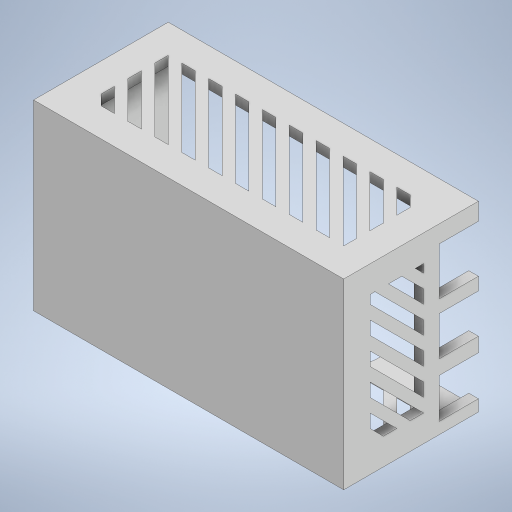
# Autodesk Inventor part: RPIcaseTop
Saved by Autodesk Inventor 2024 (Build 280153000, 153)
## iProperties
Created: 2023-07-18
Part Number: RPIcaseTop
Material: Generic
Document SubType Name: Modeling
Designer: 18179
Density: 1 g/cm^3
Appearance: Default
Autodesk Inventor part; units mm, degrees
ref_plane "YZ Plane" through (0, 0, 0) normal (1, 0, 0) x (0, 1, 0)
ref_plane "XZ Plane" through (0, 0, 0) normal (0, 1, 0) x (-1, 0, 0)
ref_plane "XY Plane" through (0, 0, 0) normal (0, 0, 1) x (1, 0, 0)
sketch "Sketch1" plane through (0, 0, 0) normal (0, 0, 1) x (1, 0, 0)
  point P0 (0, 0)
sketch "0" plane through (0, 0, 0) normal (0, 0, 1) x (1, 0, 0)
  line L0 (-14.825, -56.3549) -> (-14.825, 0.3263)
  line L1 (-14.825, 0.3263) -> (82.381, 0.3263)
  line L2 (82.381, 0.3263) -> (82.381, -2.3)
  line L3 (82.381, -2.3) -> (85.6, -2.3)
  line L4 (85.6, -2.3) -> (85.6, 3.5013)
  line L5 (85.6, 3.5013) -> (-18, 3.5013)
  line L6 (-18, 3.5013) -> (-18, -57.5)
  line L7 (-18, -57.5) -> (3.4071, -57.5)
  line L8 (3.4071, -57.5) -> (3.4071, -56.3549)
  line L9 (3.4071, -56.3549) -> (-14.825, -56.3549)
  line L10 (-14.825, -56.3549) -> (82.381, -56.3549)
  line L11 (82.381, -56.3549) -> (82.381, 0.3263)
  line L12 (82.381, 0.3263) -> (-14.825, 0.3263)
  line L13 (-14.825, 0.3263) -> (-14.825, -56.3549)
  line L14 (13.029, -57.5) -> (13.029, -56.3549)
  line L15 (13.029, -56.3549) -> (3.4071, -56.3549)
  line L16 (3.4071, -56.3549) -> (3.4071, -57.5)
  line L17 (3.4071, -57.5) -> (13.029, -57.5)
  line L18 (19.369, -56.3549) -> (13.029, -56.3549)
  line L19 (13.029, -56.3549) -> (13.029, -57.5)
  line L20 (13.029, -57.5) -> (19.369, -57.5)
  line L21 (19.369, -57.5) -> (19.369, -56.3549)
  line L22 (26.631, -57.5) -> (26.631, -56.3549)
  line L23 (26.631, -56.3549) -> (19.369, -56.3549)
  line L24 (19.369, -56.3549) -> (19.369, -57.5)
  line L25 (19.369, -57.5) -> (26.631, -57.5)
  line L26 (32.869, -56.3549) -> (26.631, -56.3549)
  line L27 (26.631, -56.3549) -> (26.631, -57.5)
  line L28 (26.631, -57.5) -> (32.869, -57.5)
  line L29 (32.869, -57.5) -> (32.869, -56.3549)
  line L30 (40.131, -57.5) -> (40.131, -56.3549)
  line L31 (40.131, -56.3549) -> (32.869, -56.3549)
  line L32 (32.869, -56.3549) -> (32.869, -57.5)
  line L33 (32.869, -57.5) -> (40.131, -57.5)
  line L34 (47.619, -56.3549) -> (40.131, -56.3549)
  line L35 (40.131, -56.3549) -> (40.131, -57.5)
  line L36 (40.131, -57.5) -> (47.619, -57.5)
  line L37 (47.619, -57.5) -> (47.619, -56.3549)
  line L38 (54.381, -57.5) -> (54.381, -56.3549)
  line L39 (54.381, -56.3549) -> (47.619, -56.3549)
  line L40 (47.619, -56.3549) -> (47.619, -57.5)
  line L41 (47.619, -57.5) -> (54.381, -57.5)
  line L42 (82.381, -56.3549) -> (54.381, -56.3549)
  line L43 (54.381, -56.3549) -> (54.381, -57.5)
  line L44 (54.381, -57.5) -> (85.6, -57.5)
  line L45 (85.6, -57.5) -> (85.6, -53.65)
  line L46 (85.6, -53.65) -> (82.381, -53.65)
  line L47 (82.381, -53.65) -> (82.381, -56.3549)
  line L48 (82.381, -53.65) -> (85.6, -53.65)
  line L49 (85.6, -53.65) -> (85.6, -40.35)
  line L50 (85.6, -40.35) -> (82.381, -40.35)
  line L51 (82.381, -40.35) -> (82.381, -53.65)
  line L52 (82.381, -35.55) -> (85.6, -35.55)
  line L53 (85.6, -35.55) -> (85.6, -22.45)
  line L54 (85.6, -22.45) -> (82.381, -22.45)
  line L55 (82.381, -22.45) -> (82.381, -35.55)
  line L56 (82.381, -18.2) -> (85.6, -18.2)
  line L57 (85.6, -18.2) -> (85.6, -2.3)
  line L58 (85.6, -2.3) -> (82.381, -2.3)
  line L59 (82.381, -2.3) -> (82.381, -18.2)
  line L60 (85.6, -18.2) -> (82.381, -18.2)
  line L61 (82.381, -18.2) -> (82.381, -22.45)
  line L62 (82.381, -22.45) -> (85.6, -22.45)
  line L63 (85.6, -22.45) -> (85.6, -18.2)
  line L64 (85.6, -40.35) -> (85.6, -35.55)
  line L65 (85.6, -35.55) -> (82.381, -35.55)
  line L66 (82.381, -35.55) -> (82.381, -40.35)
  line L67 (82.381, -40.35) -> (85.6, -40.35)
  circle A0 centre (58.5, -3.5) radius 1.35
  circle A1 centre (58.5, -52.5) radius 1.35
  circle A2 centre (0.5, -52.5) radius 1.35
  circle A3 centre (0.5, -3.5) radius 1.35
  line L68 (26.631, -57.5) -> (32.869, -57.5)
  line L69 (85.6, -18.2) -> (85.6, -2.3)
  point P0 (-14.825, 0.3263)
  point P1 (82.381, -2.3)
  point P2 (85.6, 3.5013)
  point P3 (-18, 3.5013)
  constraints: 140 end point, 4 centre point
extrude "Extrusion1" add sketch "0" along normal blind 40 contours L9 L8 L7 L6 L5 L4 L3 L2 L1 L0 | L10 L21 L20 L14 | L56 L63 L54 L11 | L10 L29 L28 L22 | L52 L64 L50 L11 | L10 L37 L36 L30 | L46 L45 L44 L38 L10 L11
sketch "Sketch3" plane through (0, 0, 40) normal (0, 0, 1) x (1, 0, 0)
  line L0 (3.4071, -57.5) -> (3.4071, -56.3549) projected
  line L1 (3.4071, -56.3549) -> (-14.825, -56.3549) projected
  line L2 (-14.825, -56.3549) -> (-14.825, 0.3263) projected
  line L3 (-14.825, 0.3263) -> (82.381, 0.3263) projected
  line L4 (82.381, 0.3263) -> (82.381, -2.3) projected
  line L5 (82.381, -2.3) -> (85.6, -2.3) projected
  line L6 (85.6, -2.3) -> (85.6, 3.5013) projected
  line L7 (85.6, 3.5013) -> (-18, 3.5013) projected
  line L8 (-18, 3.5013) -> (-18, -57.5) projected
  line L9 (-18, -57.5) -> (3.4071, -57.5) projected
  line L10 (19.369, -57.5) -> (19.369, -56.3549) projected
  line L11 (19.369, -56.3549) -> (13.029, -56.3549) projected
  line L12 (13.029, -56.3549) -> (13.029, -57.5) projected
  line L13 (13.029, -57.5) -> (19.369, -57.5) projected
  line L14 (40.131, -56.3549) -> (40.131, -57.5) projected
  line L15 (82.381, -56.3549) -> (54.381, -56.3549) projected
  line L16 (32.869, -57.5) -> (32.869, -56.3549) projected
  line L17 (85.6, -57.5) -> (85.6, -53.65) projected
  line L18 (85.6, -53.65) -> (82.381, -53.65) projected
  line L19 (82.381, -53.65) -> (82.381, -56.3549) projected
  line L20 (82.381, -56.3549) -> (54.381, -56.3549) projected
  line L21 (47.619, -57.5) -> (47.619, -56.3549) projected
  line L22 (85.6, -35.55) -> (82.381, -35.55) projected
  line L23 (82.381, -35.55) -> (82.381, -40.35) projected
  line L24 (82.381, -40.35) -> (85.6, -40.35) projected
  line L25 (85.6, -40.35) -> (85.6, -35.55) projected
  line L26 (85.6, -18.2) -> (82.381, -18.2) projected
  line L27 (82.381, -18.2) -> (82.381, -22.45) projected
  line L28 (82.381, -22.45) -> (85.6, -22.45) projected
  line L29 (85.6, -22.45) -> (85.6, -18.2) projected
  line L30 (-18, -57.5) -> (3.4071, -57.5) projected
  line L31 (3.4071, -57.5) -> (13.029, -57.5)
  line L32 (13.029, -57.5) -> (13.029, -56.3549)
  line L33 (13.029, -56.3549) -> (3.4071, -56.3549)
  line L34 (3.4071, -56.3549) -> (3.4071, -57.5)
  line L35 (19.369, -57.5) -> (32.869, -57.5)
  line L36 (32.869, -57.5) -> (32.869, -56.3549)
  line L37 (32.869, -56.3549) -> (19.369, -56.3549)
  line L38 (19.369, -56.3549) -> (19.369, -57.5)
  line L39 (40.131, -57.5) -> (47.619, -57.5)
  line L40 (47.619, -57.5) -> (47.619, -56.3549)
  line L41 (47.619, -56.3549) -> (40.131, -56.3549)
  line L42 (40.131, -56.3549) -> (40.131, -57.5)
  line L43 (85.6, -53.65) -> (82.381, -53.65)
  line L44 (82.381, -53.65) -> (82.381, -40.35)
  line L45 (82.381, -40.35) -> (85.6, -40.35)
  line L46 (85.6, -40.35) -> (85.6, -53.65)
  line L47 (85.6, -35.55) -> (82.381, -35.55)
  line L48 (82.381, -35.55) -> (82.381, -22.45)
  line L49 (82.381, -22.45) -> (85.6, -22.45)
  line L50 (85.6, -22.45) -> (85.6, -35.55)
  line L51 (85.6, -18.2) -> (82.381, -18.2)
  line L52 (82.381, -18.2) -> (82.381, -2.3)
  line L53 (82.381, -2.3) -> (85.6, -2.3)
  line L54 (85.6, -2.3) -> (85.6, -18.2)
  line L55 (47.619, -56.3549) -> (40.131, -56.3549) projected
  line L56 (40.131, -56.3549) -> (40.131, -57.5) projected
  line L57 (40.131, -57.5) -> (47.619, -57.5) projected
  line L58 (19.369, -57.5) -> (19.369, -56.3549) projected
  line L59 (19.369, -56.3549) -> (13.029, -56.3549) projected
  line L60 (13.029, -56.3549) -> (13.029, -57.5) projected
  line L61 (13.029, -57.5) -> (19.369, -57.5) projected
  line L62 (32.869, -56.3549) -> (26.631, -56.3549) projected
  line L63 (26.631, -56.3549) -> (26.631, -57.5) projected
  line L64 (26.631, -57.5) -> (32.869, -57.5) projected
  line L65 (32.869, -57.5) -> (32.869, -56.3549) projected
  line L66 (54.381, -56.3549) -> (54.381, -57.5) projected
  line L67 (54.381, -57.5) -> (85.6, -57.5) projected
  line L68 (47.619, -57.5) -> (47.619, -56.3549) projected
  line L69 (47.619, -56.3549) -> (40.131, -56.3549) projected
  line L70 (40.131, -57.5) -> (47.619, -57.5) projected
  line L71 (19.369, -57.5) -> (19.369, -56.3549) projected
  line L72 (19.369, -56.3549) -> (13.029, -56.3549) projected
  line L73 (13.029, -56.3549) -> (13.029, -57.5) projected
  line L74 (13.029, -57.5) -> (19.369, -57.5) projected
  line L75 (32.869, -56.3549) -> (26.631, -56.3549) projected
  line L76 (26.631, -56.3549) -> (26.631, -57.5) projected
  line L77 (26.631, -57.5) -> (32.869, -57.5) projected
  line L78 (85.6, -53.65) -> (82.381, -53.65) projected
  line L79 (82.381, -53.65) -> (82.381, -56.3549) projected
  line L80 (54.381, -56.3549) -> (54.381, -57.5) projected
  line L81 (54.381, -57.5) -> (85.6, -57.5) projected
  line L82 (85.6, -57.5) -> (85.6, -53.65) projected
  point P0 (0, 0)
  constraints: 48 end point, 12 parallel, 6 horizontal, 6 perpendicular
extrude "Extrusion2" add sketch "Sketch3" against normal blind 26.919 contours L54 L26 L52 L5 | L50 L22 L48 L28 | L46 L18 L44 L24
sketch "Sketch6" plane through (0, 0, 40) normal (0, 0, 1) x (1, 0, 0)
  line L0 (54.381, -56.3549) -> (54.381, -57.5) projected
  line L1 (47.619, -56.3549) -> (40.131, -56.3549) projected
  line L2 (54.381, -57.5) -> (47.619, -57.5)
  line L3 (47.619, -57.5) -> (47.619, -56.3549)
  line L4 (47.619, -56.3549) -> (54.381, -56.3549)
  line L5 (54.381, -56.3549) -> (54.381, -57.5)
  point P0 (0, 0)
  constraints: 8 end point, 2 parallel, 1 horizontal, 1 perpendicular
extrude "Extrusion4" add sketch "Sketch6" against normal blind 33.2436
fillet "Fillet2" radius 3.175 2 edges at (47.619, -56.9275, 6.7564) (54.381, -56.9275, 6.7564)
sketch "Sketch7" plane through (0, 0, 40) normal (0, 0, 1) x (1, 0, 0)
  line L0 (3.4071, -57.5) -> (3.4071, -56.3549) projected
  line L1 (13.029, -57.5) -> (19.369, -57.5) projected
  line L2 (3.4071, -56.3549) -> (13.029, -56.3549)
  line L3 (13.029, -56.3549) -> (13.029, -57.5)
  line L4 (13.029, -57.5) -> (3.4071, -57.5)
  line L5 (3.4071, -57.5) -> (3.4071, -56.3549)
  line L6 (19.369, -57.5) -> (19.369, -56.3549) projected
  line L7 (26.631, -56.3549) -> (26.631, -57.5) projected
  line L8 (19.369, -56.3549) -> (26.631, -56.3549)
  line L9 (26.631, -56.3549) -> (26.631, -57.5)
  line L10 (26.631, -57.5) -> (19.369, -57.5)
  line L11 (19.369, -57.5) -> (19.369, -56.3549)
  line L12 (32.869, -57.5) -> (32.869, -56.3549) projected
  line L13 (40.131, -56.3549) -> (40.131, -57.5) projected
  line L14 (32.869, -56.3549) -> (40.131, -56.3549)
  line L15 (40.131, -56.3549) -> (40.131, -57.5)
  line L16 (40.131, -57.5) -> (32.869, -57.5)
  line L17 (32.869, -57.5) -> (32.869, -56.3549)
  point P0 (0, 0)
  constraints: 24 end point, 6 parallel, 3 horizontal, 3 perpendicular
extrude "Extrusion5" add sketch "Sketch7" against normal blind 36.8504
fillet "Fillet3" radius 1.524 2 edges at (3.4071, -56.9275, 3.1496) (13.029, -56.9275, 3.1496)
fillet "Fillet4" radius 0.762 4 edges at (19.369, -56.9275, 3.1496) (26.631, -56.9275, 3.1496) (32.869, -56.9275, 3.1496) (40.131, -56.9275, 3.1496)
sketch "Sketch8" plane through (0, 0, 40) normal (0, 0, 1) x (1, 0, 0)
  line L0 (-14.825, -56.3549) -> (-14.825, 0.3263) projected
  line L1 (-14.825, 0.3263) -> (82.381, 0.3263) projected
  line L2 (82.381, 0.3263) -> (82.381, -56.3549) projected
  line L3 (82.381, -56.3549) -> (-14.825, -56.3549) projected
  point P0 (0, 0)
extrude "Extrusion6" add sketch "Sketch8" against normal blind 2
sketch "Sketch9" plane through (0, 0, 40) normal (0, 0, 1) x (1, 0, 0)
  line L0 (-18, -57.5) -> (85.6, -57.5) projected
  line L1 (85.6, -57.5) -> (85.6, 3.5013) projected
  line L2 (85.6, 3.5013) -> (-18, 3.5013) projected
  line L3 (-18, 3.5013) -> (-18, -57.5) projected
  point P0 (0, 0)
extrude "Extrusion7" add sketch "Sketch9" along normal blind 5
sketch "Sketch10" plane through (54.381, -57.5, 0) normal (0, -1, 0) x (1, 0, 0)
  line L0 (-27.75, 0) -> (-21.512, 0) projected
  line L1 (-21.512, 0) -> (-21.512, 2.3876) projected
  arc A0 (-20.75, 3.1496) -> (-21.512, 2.3876) centre (-20.75, 2.3876) ccw projected
  line L2 (-15.012, 3.1496) -> (-20.75, 3.1496) projected
  arc A1 (-14.25, 2.3876) -> (-15.012, 3.1496) centre (-15.012, 2.3876) ccw projected
  line L3 (-14.25, 0) -> (-14.25, 2.3876) projected
  line L4 (-14.25, 0) -> (-6.762, 0) projected
  line L5 (-6.762, 0) -> (-6.762, 3.5814) projected
  arc A2 (-3.587, 6.7564) -> (-6.762, 3.5814) centre (-3.587, 3.5814) ccw projected
  line L6 (-3.175, 6.7564) -> (-3.587, 6.7564) projected
  arc A3 (0, 3.5814) -> (-3.175, 6.7564) centre (-3.175, 3.5814) ccw projected
  line L7 (0, 0) -> (0, 3.5814) projected
  line L8 (0, 0) -> (31.219, 0) projected
  line L9 (31.219, 0) -> (31.219, 45) projected
  line L10 (-72.381, 45) -> (31.219, 45) projected
  line L11 (-72.381, 0) -> (-72.381, 45) projected
  line L12 (-72.381, 0) -> (-50.9739, 0) projected
  line L13 (-50.9739, 0) -> (-50.9739, 1.6256) projected
  arc A4 (-49.4499, 3.1496) -> (-50.9739, 1.6256) centre (-49.4499, 1.6256) ccw projected
  line L14 (-42.876, 3.1496) -> (-49.4499, 3.1496) projected
  arc A5 (-41.352, 1.6256) -> (-42.876, 3.1496) centre (-42.876, 1.6256) ccw projected
  line L15 (-41.352, 0) -> (-41.352, 1.6256) projected
  line L16 (-41.352, 0) -> (-35.012, 0) projected
  line L17 (-35.012, 0) -> (-35.012, 2.3876) projected
  arc A6 (-34.25, 3.1496) -> (-35.012, 2.3876) centre (-34.25, 2.3876) ccw projected
  line L18 (-28.512, 3.1496) -> (-34.25, 3.1496) projected
  arc A7 (-27.75, 2.3876) -> (-28.512, 3.1496) centre (-28.512, 2.3876) ccw projected
  line L19 (-27.75, 0) -> (-27.75, 2.3876) projected
  line L20 (36.8849, 50.6659) -> (36.8849, -5.6659)
  line L21 (36.8849, -5.6659) -> (-1.0961, -5.6659)
  line L22 (-1.0961, -5.6659) -> (-15.8461, -5.6659)
  line L23 (-15.8461, -5.6659) -> (-29.3461, -5.6659)
  line L24 (-29.3461, -5.6659) -> (-45.3079, -5.6659)
  line L25 (-45.3079, -5.6659) -> (-78.0469, -5.6659)
  line L26 (-78.0469, -5.6659) -> (-78.0469, 50.6659)
  line L27 (-78.0469, 50.6659) -> (36.8849, 50.6659)
  line L28 (21.6449, 35.4259) -> (21.6449, 9.5741)
  line L29 (21.6449, 9.5741) -> (-1.0961, 9.5741)
  line L30 (-1.0961, 9.5741) -> (-15.8461, 9.5741)
  line L31 (-15.8461, 9.5741) -> (-29.3461, 9.5741)
  line L32 (-29.3461, 9.5741) -> (-45.3079, 9.5741)
  line L33 (-45.3079, 9.5741) -> (-62.8069, 9.5741)
  line L34 (-62.8069, 9.5741) -> (-62.8069, 35.4259)
  line L35 (-62.8069, 35.4259) -> (21.6449, 35.4259)
  line L36 (-62.8069, 9.5741) -> (-34.25, 38.131)
  line L37 (-62.8069, 9.5741) -> (-22.4213, 9.5741) construction
  line L38 (-60.5619, 7.329) -> (-32.0049, 35.8859)
  line L39 (-58.3168, 5.0839) -> (-29.7599, 33.6409)
  line L40 (-65.052, 11.8191) -> (-36.4951, 40.3761)
  line L41 (-67.2971, 14.0642) -> (-38.7401, 42.6211)
  line L42 (-69.5421, 16.3092) -> (-40.9852, 44.8662)
  line L43 (-71.7872, 18.5543) -> (-43.2303, 47.1113)
  line L44 (-74.0323, 20.7994) -> (-45.4753, 49.3563)
  line L45 (-56.0718, 2.8389) -> (-27.5148, 31.3958)
  line L46 (-53.8267, 0.5938) -> (-25.2697, 29.1507)
  line L47 (-51.5816, -1.6513) -> (-23.0247, 26.9057)
  line L48 (-49.3366, -3.8963) -> (-20.7796, 24.6606)
  line L49 (-47.0915, -6.1414) -> (-18.5346, 22.4156)
  line L50 (-44.8464, -8.3865) -> (-16.2895, 20.1705)
  line L51 (-16.2895, 20.1705) -> (-1.034, 35.4259)
  line L52 (1.211, 33.1809) -> (-14.0444, 17.9254)
  line L53 (-14.0444, 17.9254) -> (-42.6014, -10.6315)
  line L54 (-1.034, 35.4259) -> (-16.2895, 20.1705)
  line L55 (-16.2895, 20.1705) -> (-44.8464, -8.3865)
  line L56 (3.4561, 30.9358) -> (-11.7994, 15.6804)
  line L57 (-11.7994, 15.6804) -> (-40.3563, -12.8766)
  line L58 (5.7012, 28.6908) -> (-9.5543, 13.4353)
  line L59 (-9.5543, 13.4353) -> (-38.1112, -15.1217)
  line L60 (7.9462, 26.4457) -> (-7.3092, 11.1902)
  line L61 (-7.3092, 11.1902) -> (-35.8662, -17.3667)
  line L62 (10.1913, 24.2006) -> (-5.0642, 8.9452)
  line L63 (-5.0642, 8.9452) -> (-33.6211, -19.6118)
  line L64 (12.4364, 21.9556) -> (-2.8191, 6.7001)
  line L65 (-2.8191, 6.7001) -> (-31.3761, -21.8568)
  line L66 (14.6814, 19.7105) -> (-0.574, 4.455)
  line L67 (-0.574, 4.455) -> (-29.131, -24.1019)
  line L68 (16.9265, 17.4654) -> (1.671, 2.21)
  line L69 (1.671, 2.21) -> (-26.8859, -26.347)
  line L70 (19.1715, 15.2204) -> (3.9161, -0.0351)
  line L71 (3.9161, -0.0351) -> (-24.6409, -28.592)
  line L72 (21.4166, 12.9753) -> (6.1612, -2.2802)
  line L73 (6.1612, -2.2802) -> (-22.3958, -30.8371)
  line L74 (-29.7599, 33.6409) -> (-26.8859, 36.5148)
  line L75 (-27.5148, 31.3958) -> (-22.3958, 36.5148)
  line L76 (-25.2697, 29.1507) -> (-14.0444, 40.3761)
  line L77 (-23.0247, 26.9057) -> (-2.8191, 47.1113)
  line L78 (-20.7796, 24.6606) -> (1.671, 47.1113)
  line L79 (-18.5346, 22.4156) -> (6.1612, 47.1113)
  line L80 (1.211, 33.1809) -> (3.4561, 35.4259)
  line L81 (3.4561, 30.9358) -> (20.3918, 47.8715)
  line L82 (5.7012, 28.6908) -> (12.4364, 35.4259)
  line L83 (7.9462, 26.4457) -> (16.9265, 35.4259)
  line L84 (10.1913, 24.2006) -> (21.6449, 35.6543)
  line L85 (12.4364, 21.9556) -> (21.6449, 31.1642)
  line L86 (14.6814, 19.7105) -> (21.6449, 26.674)
  line L87 (16.9265, 17.4654) -> (21.6449, 22.1839)
  line L88 (19.1715, 15.2204) -> (22.7691, 18.818)
  line L89 (21.4166, 12.9753) -> (21.6449, 13.2036)
  point P0 (-54.381, 0)
  point P1 (21.6449, 17.6938)
  point P2 (13.5252, 9.5741)
  point P3 (18.0154, 9.5741)
  point P4 (4.545, 9.5741)
  point P5 (9.0351, 9.5741)
  point P6 (21.4166, 35.4259)
  point P7 (-4.4353, 9.5741)
  point P8 (0.0548, 9.5741)
  point P9 (-13.4155, 9.5741)
  point P10 (-8.9254, 9.5741)
  point P11 (-22.3958, 9.5741)
  point P12 (-17.9057, 9.5741)
  point P13 (7.9462, 35.4259)
  point P14 (-5.5242, 35.4259)
  point P15 (-31.3761, 9.5741)
  point P16 (-26.8859, 9.5741)
  point P17 (-10.0143, 35.4259)
  point P18 (-14.5044, 35.4259)
  point P19 (-40.3563, 9.5741)
  point P20 (-35.8662, 9.5741)
  point P21 (-18.9945, 35.4259)
  point P22 (-23.4847, 35.4259)
  point P23 (-49.3366, 9.5741)
  point P24 (-44.8464, 9.5741)
  point P25 (-27.9748, 35.4259)
  point P26 (-32.4649, 35.4259)
  point P27 (-58.3168, 9.5741)
  point P28 (-53.8267, 9.5741)
  point P29 (-41.4452, 35.4259)
  point P30 (-62.8069, 14.0642)
  point P31 (-36.9551, 35.4259)
  point P32 (-50.4254, 35.4259)
  point P33 (-62.8069, 23.0444)
  point P34 (-62.8069, 18.5543)
  point P35 (-45.9353, 35.4259)
  point P36 (-59.4057, 35.4259)
  point P37 (-62.8069, 32.0247)
  point P38 (-62.8069, 27.5346)
  point P39 (-54.9156, 35.4259)
  dimension "d19" = 15.24
  dimension "d20" = 45
  dimension "d21" = 3.175
  dimension "d22" = 3.175
  dimension "d23" = 3.175
  dimension "d24" = 3.175
  dimension "d25" = 3.175
  dimension "d26" = 3.175
  dimension "d27" = 3.175
  dimension "d28" = 3.175
  dimension "d29" = 3.175
  dimension "d30" = 3.175
  dimension "d31" = 3.175
  dimension "d32" = 3.175
  dimension "d33" = 3.175
  dimension "d34" = 3.175
  dimension "d35" = 3.175
  dimension "d36" = 3.175
  dimension "d37" = 3.175
  dimension "d38" = 3.175
  dimension "d39" = 3.175
  dimension "d40" = 3.175
  dimension "d41" = 3.175
  dimension "d42" = 3.175
  dimension "d43" = 3.175
  dimension "d44" = 3.175
  constraints: 138 end point, 21 parallel, 5 point on line, 1 equal length, 1 horizontal, 32 other
  measures "d20" angle of L37 L36
  measures "d21" distance between parallel lines of L36 L38
  measures "d22" distance between parallel lines of L38 L39
  measures "d23" distance between parallel lines of L36 L40
  measures "d24" distance between parallel lines of L40 L41
  measures "d25" distance between parallel lines of L41 L42
  measures "d26" distance between parallel lines of L42 L43
  measures "d27" distance between parallel lines of L43 L44
  measures "d28" distance between parallel lines of L39 L45
  measures "d29" distance between parallel lines of L45 L46
  measures "d30" distance between parallel lines of L46 L47
  measures "d31" distance between parallel lines of L47 L48
  measures "d32" distance between parallel lines of L48 L49
  measures "d33" distance between parallel lines of L49 L50
  measures "d34" distance between parallel lines of L51 L52
  measures "d35" distance between parallel lines of L52 L54
  measures "d36" distance between parallel lines of L52 L56
  measures "d37" distance between parallel lines of L56 L58
  measures "d38" distance between parallel lines of L58 L60
  measures "d39" distance between parallel lines of L60 L62
  measures "d40" distance between parallel lines of L62 L64
  measures "d41" distance between parallel lines of L64 L66
  measures "d42" distance between parallel lines of L66 L68
  measures "d43" distance between parallel lines of L68 L70
  measures "d44" distance between parallel lines of L70 L72
extrude "Extrusion8" cut sketch "Sketch10" against normal through all contours L31 L53 L52 L80 L35 L81 L56 L57 | L59 L58 L82 L35 L83 L60 L61 L30 | L31 L32 L49 L79 L35 L51 L50 | L62 L84 L35 L28 L85 L64 L29 L30 | L32 L47 L77 L35 L78 L48 | L66 L86 L28 L87 L68 L29 | L32 L33 L45 L75 L35 L76 L46 | L29 L70 L88 L28 L89 L72 | L43 L34 L44 L35 | L33 L38 L35 L74 L39 | L35 L41 L34 L42 | L34 L40 L35 L36
sketch "Sketch11" plane through (85.6, -2.3, 0) normal (1, 0, 0) x (0, 0, -1)
  line L0 (0, 5.8013) -> (-45, 5.8013) projected
  line L1 (-45, 5.8013) -> (-13.081, 5.8013)
  line L2 (-13.2036, 2.6263) -> (-13.2036, 5.8013) projected
  line L3 (-13.2036, 5.8013) -> (-45, 5.8013)
  line L4 (-45, 5.8013) -> (-45, -55.2)
  line L5 (-45, -55.2) -> (-13.2036, -55.2)
  line L6 (-13.2036, -55.2) -> (-13.2036, 5.8013)
  line L7 (-36.11, -46.31) -> (-36.11, -3.0887)
  line L8 (-36.11, -3.0887) -> (-22.0936, -3.0887)
  line L9 (-22.0936, -3.0887) -> (-22.0936, -46.31) construction
  line L10 (-22.0936, -46.31) -> (-36.11, -46.31)
  line L11 (-22.0936, -46.31) -> (-18.2836, -46.31)
  line L12 (-18.2836, -46.31) -> (-18.2836, -3.0887)
  line L13 (-18.2836, -3.0887) -> (-22.0936, -3.0887)
  line L14 (-22.0936, -3.0887) -> (-22.0936, -46.31) construction
  line L15 (-18.2836, -46.31) -> (-36.11, -28.4836)
  line L16 (-18.2836, -46.31) -> (6.9266, -46.31) construction
  line L17 (-16.0386, -44.0649) -> (-33.8649, -26.2386)
  line L18 (-13.7935, -41.8199) -> (-31.6199, -23.9935)
  line L19 (-11.5485, -39.5748) -> (-29.3748, -21.7485)
  line L20 (-9.3034, -37.3297) -> (-27.1297, -19.5034)
  line L21 (-7.0583, -35.0847) -> (-24.8847, -17.2583)
  line L22 (-4.8133, -32.8396) -> (-22.6396, -15.0133)
  line L23 (-22.6396, -15.0133) -> (-40.2791, 2.6263)
  line L24 (-42.5242, 0.3812) -> (-24.8847, -17.2583)
  line L25 (-24.8847, -17.2583) -> (-7.0583, -35.0847)
  line L26 (-44.7693, -1.8639) -> (-27.1297, -19.5034)
  line L27 (-27.1297, -19.5034) -> (-9.3034, -37.3297)
  line L28 (-47.0143, -4.1089) -> (-29.3748, -21.7485)
  line L29 (-29.3748, -21.7485) -> (-11.5485, -39.5748)
  line L30 (-49.2594, -6.354) -> (-31.6199, -23.9935)
  line L31 (-31.6199, -23.9935) -> (-13.7935, -41.8199)
  line L32 (-51.5044, -8.5991) -> (-33.8649, -26.2386)
  line L33 (-33.8649, -26.2386) -> (-16.0386, -44.0649)
  line L34 (-38.0341, 4.8713) -> (-20.3946, -12.7682)
  line L35 (-20.3946, -12.7682) -> (-2.5682, -30.5946)
  line L36 (-35.789, 7.1164) -> (-18.1495, -10.5231)
  line L37 (-18.1495, -10.5231) -> (-0.3231, -28.3495)
  line L38 (-33.5439, 9.3614) -> (-15.9044, -8.2781)
  line L39 (-15.9044, -8.2781) -> (1.9219, -26.1044)
  line L40 (-20.5287, -48.5551) -> (-38.3551, -30.7287)
  line L41 (-18.2836, -46.31) -> (-36.11, -28.4836)
  line L42 (-22.7738, -50.8001) -> (-40.6001, -32.9738)
  line L43 (-25.0188, -53.0452) -> (-42.8452, -35.2188)
  point P0 (0, 2.3)
  point P1 (-13.081, 0)
  point P2 (-21.0937, -3.0887)
  point P3 (-18.2836, -5.8988)
  point P4 (-18.2836, -10.389)
  point P5 (-25.5839, -3.0887)
  point P6 (-30.074, -3.0887)
  point P7 (-18.2836, -14.8791)
  point P8 (-36.11, -6.033)
  point P9 (-18.2836, -23.8594)
  point P10 (-18.2836, -19.3692)
  point P11 (-34.5641, -3.0887)
  point P12 (-36.11, -15.0133)
  point P13 (-18.2836, -32.8396)
  point P14 (-18.2836, -28.3495)
  point P15 (-27.1297, -19.5034)
  point P16 (-36.11, -10.5231)
  point P17 (-36.11, -23.9935)
  point P18 (-18.2836, -41.8199)
  point P19 (-18.2836, -37.3297)
  point P20 (-36.11, -19.5034)
  point P21 (-36.11, -32.9738)
  point P22 (-22.7738, -46.31)
  point P23 (-36.11, -41.954)
  point P24 (-31.754, -46.31)
  point P25 (-27.2639, -46.31)
  point P26 (-36.11, -37.4639)
  dimension "d61" = 8.89
  dimension "d62" = 3.81
  dimension "d63" = 135
  dimension "d64" = 3.175
  dimension "d65" = 3.175
  dimension "d66" = 3.175
  dimension "d67" = 3.175
  dimension "d68" = 3.175
  dimension "d69" = 3.175
  dimension "d70" = 3.175
  dimension "d71" = 3.175
  dimension "d72" = 3.175
  dimension "d73" = 3.175
  dimension "d74" = 3.175
  dimension "d75" = 3.175
  dimension "d76" = 3.175
  dimension "d77" = 3.175
  dimension "d78" = 3.175
  dimension "d79" = 3.175
  dimension "d80" = 3.175
  dimension "d81" = 3.175
  constraints: 84 end point, 16 parallel, 3 horizontal, 3 perpendicular, 1 equal length, 1 point on line, 11 other
  measures "d61" distance between parallel lines of L4 L7
  measures "d62" distance of L13.end L12.end
  measures "d63" angle of L16 L15
  measures "d64" distance between parallel lines of L15 L17
  measures "d65" distance between parallel lines of L17 L18
  measures "d66" distance between parallel lines of L18 L19
  measures "d67" distance between parallel lines of L19 L20
  measures "d68" distance between parallel lines of L20 L21
  measures "d69" distance between parallel lines of L21 L22
  measures "d70" distance between parallel lines of L23 L24
  measures "d71" distance between parallel lines of L24 L26
  measures "d72" distance between parallel lines of L26 L28
  measures "d73" distance between parallel lines of L28 L30
  measures "d74" distance between parallel lines of L30 L32
  measures "d75" distance between parallel lines of L23 L34
  measures "d76" distance between parallel lines of L34 L36
  measures "d77" distance between parallel lines of L36 L38
  measures "d78" distance between parallel lines of L15 L40
  measures "d79" distance between parallel lines of L40 L41
  measures "d80" distance between parallel lines of L40 L42
  measures "d81" distance between parallel lines of L42 L43
extrude "Extrusion9" cut sketch "Sketch11" against normal blind 25.4 contours L13 L12 L38 | L36 L12 L35 L34 L8 | L7 L26 L20 L12 L19 L28 | L23 L22 L12 L21 L24 L7 L8 | L30 L18 L12 L17 L32 L7 | L15 L11 L10 L40 L7 | L42 L10 L43 L7
sketch "Sketch12" plane through (0, 0, 38) normal (0, 0, -1) x (-1, 0, 0)
  line L0 (-82.381, -53.65) -> (-82.381, -56.3549) projected
  line L1 (-82.381, 0.3263) -> (14.825, 0.3263) projected
  line L2 (-82.381, -56.3549) -> (14.825, -56.3549)
  line L3 (14.825, -56.3549) -> (14.825, 0.3263)
  line L4 (14.825, 0.3263) -> (-82.381, 0.3263)
  line L5 (-82.381, 0.3263) -> (-82.381, -56.3549)
  point P0 (0, 0)
  constraints: 8 end point, 2 parallel, 1 horizontal, 1 perpendicular
body "Solid1"
